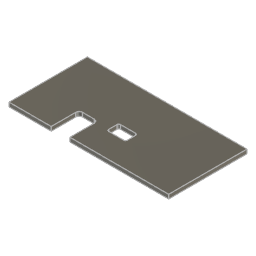
PCB Front Panel (Autodesk Fusion 360 design; units mm, degrees)
part number: 2026-07-12-16-58-24-153
Autodesk Fusion 360 part; units mm, degrees
sketch "Sketch1" plane through (0, 0, 0) normal (0, 0, 1) x (1, 0, 0)
  line L0 (-47.25, 23.2) -> (47.25, 23.2)
  line L1 (47.25, 23.2) -> (47.25, -23.2)
  line L2 (47.25, -23.2) -> (-47.25, -23.2)
  line L3 (-47.25, -23.2) -> (-47.25, 23.2)
  line L4 (-47.25, 23.2) -> (47.25, -23.2) construction
  line L5 (47.25, 23.2) -> (-47.25, -23.2) construction
  dimension "d1" = 94.5
  dimension "d2" = 46.4
  constraint horizontal L0
  constraint perpendicular L0 L1
  constraint parallel L0 L2
  constraint parallel L1 L3
  constraint coincident L4 origin
  constraint coincident L5 origin
  measures "d1" distance of L0.start L0.end
  measures "d2" distance of L0.start L2.end
extrude "Extrude1" add sketch "Sketch1" along normal blind 2.5
sketch "Sketch2" plane through (0, 0, 2.5) normal (0, 0, 1) x (-1, 0, 0)
  line L0 (47.25, 23.2) -> (-47.25, 23.2)
  line L1 (-47.25, 23.2) -> (-47.25, -23.2)
  line L2 (-47.25, -23.2) -> (47.25, -23.2)
  line L3 (47.25, -23.2) -> (47.25, 23.2)
  line L4 (22.25, 6.7) -> (11.25, 6.7)
  line L5 (11.25, 6.7) -> (11.25, 23.2)
  line L6 (11.25, 23.2) -> (22.25, 23.2)
  line L7 (22.25, 23.2) -> (22.25, 6.7)
  line L8 (3.75, 1.7) -> (-7.25, 1.7)
  line L9 (-7.25, 1.7) -> (-7.25, 8.7)
  line L10 (-7.25, 8.7) -> (3.75, 8.7)
  line L11 (3.75, 8.7) -> (3.75, 1.7)
  dimension "d5" = 11
  dimension "d6" = 16.5
  dimension "d7" = 25
  dimension "d12" = 21.5
  dimension "d13" = 40
  dimension "d14" = 11
  dimension "d15" = 7
  constraint horizontal L4
  constraint vertical L5
  constraint horizontal L6
  constraint vertical L7
  constraint collinear L0 L6
  constraint horizontal L8
  constraint vertical L9
  constraint horizontal L10
  constraint vertical L11
  measures "d5" distance of L4.start L4.end
  measures "d6" distance of L4.start L6.end
  measures "d7" distance of L3 L7
  measures "d12" distance of L0 L8
  measures "d13" distance of L1 L9
  measures "d14" distance of L8.start L8.end
  measures "d15" distance of L8.end L9.end
extrude "Extrude2" cut sketch "Sketch2" against normal blind 5 contours L0 L4 L5 L6 L7 | L8 L9 L10 L11
fillet "Fillet1" radius 2 2 edges at (-22.25, -6.7, 1.25) (-11.25, -6.7, 1.25)
fillet "Fillet2" radius 1 4 edges at (7.25, -1.7, 1.25) (-3.75, -1.7, 1.25) (-3.75, -8.7, 1.25) (7.25, -8.7, 1.25)
sketch "Sketch3" plane through (0, 0, 2.5) normal (0, 0, 1) x (-1, 0, 0)
  line L0 (11.25, 8.7) -> (11.25, 23.2)
  line L1 (11.25, 23.2) -> (-47.25, 23.2)
  line L2 (-47.25, 23.2) -> (-47.25, -23.2)
  line L3 (-47.25, -23.2) -> (47.25, -23.2)
  line L4 (47.25, -23.2) -> (47.25, 23.2)
  line L5 (47.25, 23.2) -> (22.25, 23.2)
  line L6 (22.25, 23.2) -> (22.25, 8.7)
  arc A0 (20.25, 6.7) -> (22.25, 8.7) centre (20.25, 8.7) ccw
  line L7 (20.25, 6.7) -> (13.25, 6.7)
  arc A1 (11.25, 8.7) -> (13.25, 6.7) centre (13.25, 8.7) ccw
  line L8 (-7.25, 2.7) -> (-7.25, 7.7)
  arc A2 (-6.25, 8.7) -> (-7.25, 7.7) centre (-6.25, 7.7) ccw
  line L9 (-6.25, 8.7) -> (2.75, 8.7)
  arc A3 (3.75, 7.7) -> (2.75, 8.7) centre (2.75, 7.7) ccw
  line L10 (3.75, 7.7) -> (3.75, 2.7)
  arc A4 (2.75, 1.7) -> (3.75, 2.7) centre (2.75, 2.7) ccw
  line L11 (2.75, 1.7) -> (-6.25, 1.7)
  arc A5 (-7.25, 2.7) -> (-6.25, 1.7) centre (-6.25, 2.7) ccw
  line L12 (-7.25, 5.2) -> (-7.25, 2.7)
  constraint midpoint L8 L12.start
  constraint coincident L8.start A5.start
equation "d2 = 52.65 mm - 6.25 mm"
